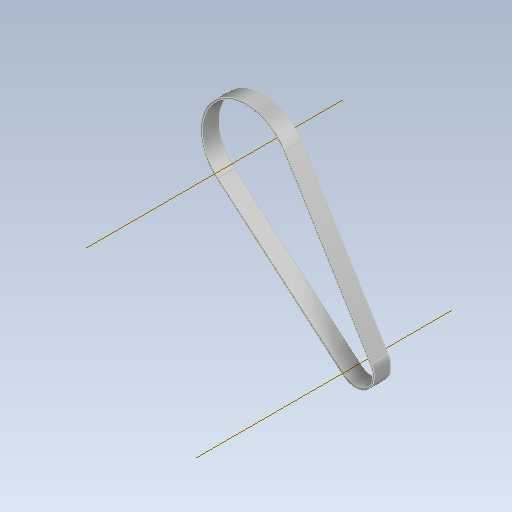
# Autodesk Inventor part: Зубчатый ремень
Saved by Autodesk Inventor 2021 (Build 250183000, 183)
## iProperties
Created: 2021-06-15
Part Number: Зубчатый ремень
Material: Rubber
Document SubType Name: Modeling
Designer: panda
Density: 1 g/cm^3
Appearance: Rubber - Black - Version 1.1
CustomPartVersion: 1
Author: panda
Autodesk Inventor part; units mm, degrees
sketch "Эскизная траектория" plane through (0, 0, 0) normal (0, 0, 1) x (1, 0, 0)
  arc A0 (156.9447, -115.4308) -> (187.2295, -89.4313) centre (170, -100) ccw
  arc A1 (88.4854, 71.545) -> (12.7733, 6.5462) centre (45.4117, 45.1233) ccw
  line L0 (88.4854, 71.545) -> (187.2295, -89.4313)
  line L1 (156.9447, -115.4308) -> (12.7733, 6.5462)
  constraints: 4 end point, 4 point on circle, 2 centre point
ref_plane "Плоскость сечения" through (187.2295, -89.4313, 0) normal (-0.5229, 0.8524, 0) x (0, 0, 1)
ref_plane "РабПлоскость2" through (170, -100, 0) normal (-1, 0, 0) x (0, 0, 1)
ref_plane "РабПлоскость3" through (45.4117, 45.1233, 0) normal (0.7614, -0.6483, 0) x (0, 0, 1)
sketch "Сечение" plane through (187.2295, -89.4313, 0) normal (-0.5229, 0.8524, 0) x (0, 0, 1)
  line L0 (-9.525, 1.3462) -> (9.525, 1.3462)
  line L1 (9.525, 1.3462) -> (9.525, -0.6858)
  line L2 (9.525, -0.6858) -> (-9.525, -0.6858)
  line L3 (-9.525, -0.6858) -> (-9.525, 1.3462)
  line L4 (-9.525, 0) -> (9.525, 0) construction
  point P0 (0, 0)
  point P1 (0, 0)
  dimension "d0" = 19.05
  dimension "d4" = 0.6858
  dimension "d5" = 1.3462
  constraints: 10 end point, 2 parallel, 2 point on line, 1 coincident, 1 horizontal, 1 midpoint, 1 perpendicular, 1 other
  measures "d0" distance between parallel lines of L1 L3
  measures "d4" distance between parallel lines of L2 L4
  measures "d5" distance between parallel lines of L4 L0
sweep "Ремень" add profiles "Сечение" path "Эскизная траектория"
equation "\"d0\" = da_B"
equation "\"d4\" = da_a"
equation "\"d5\" = da_a2"
equation "\"da_B\" = 19.05"
equation "\"da_pb\" = 12.7"
equation "\"da_L\" = 609.6"
equation "\"da_a\" = 0.6858"
equation "\"da_S\" = 6.1214"
equation "\"da_Beta\" = 20deg"
equation "\"da_Ht\" = 2.286"
equation "\"da_H\" = 4.318"
equation "\"da_a2\" = 1.3462"
body "Solid1"
